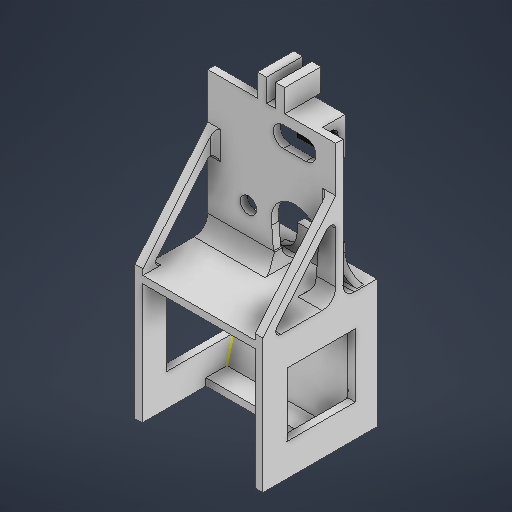
# Autodesk Inventor part: ведро
Saved by Autodesk Inventor 2025 (Build 290162000, 162)
## iProperties
Created: 2025-01-14
Part Number: ведро
Material: Типовые
Document SubType Name: Modeling
Designer: Phantom
Density: 1 g/cm^3
Appearance: По умолчанию
Author: Phantom
Autodesk Inventor part; units mm, degrees
ref_plane "YZ Plane" through (0, 0, 0) normal (1, 0, 0) x (0, 1, 0)
ref_plane "XZ Plane" through (0, 0, 0) normal (0, 1, 0) x (-1, 0, 0)
ref_plane "XY Plane" through (0, 0, 0) normal (0, 0, 1) x (1, 0, 0)
sketch "Эскиз9" plane through (0, 0, 0) normal (0, 0, 1) x (1, 0, 0)
  line L0 (-25, -25) -> (25, -25)
  line L1 (25, -25) -> (25, 25)
  line L2 (25, 25) -> (-25, 25)
  line L3 (-25, 25) -> (-25, -25)
  line L4 (-25, -25) -> (25, 25) construction
  line L5 (25, -25) -> (-25, 25) construction
  point P0 (0, 0)
  dimension "d29" = 50
  dimension "d30" = 50
  constraints: 12 end point, 2 midpoint, 2 parallel, 1 horizontal, 1 perpendicular
  measures "d29" distance of L2.end L1.end
  measures "d30" distance of L1.end L0.end
extrude "Выдавливание9" add sketch "Эскиз9" along normal blind 3.2
sketch "Эскиз10" plane through (0, 0, 0) normal (0, 0, -1) x (-1, 0, 0)
  line L0 (28.2, 28.2) -> (-28.2, 28.2)
  line L1 (-28.2, 28.2) -> (-28.2, -28.2)
  line L2 (-28.2, -28.2) -> (28.2, -28.2)
  line L3 (28.2, -28.2) -> (28.2, 28.2)
  line L4 (28.2, 28.2) -> (-28.2, -28.2) construction
  line L5 (-28.2, 28.2) -> (28.2, -28.2) construction
  line L6 (-25, -25) -> (-25, 25) projected
  line L7 (25, -25) -> (-25, -25) projected
  line L8 (25, 25) -> (25, -25) projected
  line L9 (-25, 25) -> (25, 25) projected
  point P0 (0, 0)
  dimension "d33" = 56.4
  dimension "d34" = 56.4
  constraints: 12 end point, 2 midpoint, 2 parallel, 1 horizontal, 1 perpendicular
  measures "d33" distance of L2.end L1.end
  measures "d34" distance of L1.end L0.end
extrude "Выдавливание10" add sketch "Эскиз10" against normal blind 47.2
sketch "Эскиз11" plane through (-28.2, -28.2, 0) normal (-1, 0, 0) x (0, 0, 1)
  line L0 (0, 56.4) -> (47.2, 56.4) projected
  line L1 (23.6, 56.4) -> (23.6, 0)
  line L2 (0, 0) -> (47.2, 0) projected
  line L3 (47.2, 53.2) -> (47.2, 3.2) projected
  line L4 (47.2, 28.2) -> (0, 28.2)
  line L5 (7.6, 42.2) -> (39.6, 42.2)
  line L6 (39.6, 42.2) -> (39.6, 14.2)
  line L7 (39.6, 14.2) -> (7.6, 14.2)
  line L8 (7.6, 14.2) -> (7.6, 42.2)
  line L9 (7.6, 42.2) -> (39.6, 14.2) construction
  line L10 (39.6, 42.2) -> (7.6, 14.2) construction
  line L11 (7.6, 42.2) -> (9.6, 42.2)
  line L12 (9.6, 42.2) -> (9.6, 0)
  point P0 (23.6, 28.2)
  point P1 (9.6, 14.2)
  dimension "d37" = 32
  dimension "d38" = 28
  dimension "d51" = 2
  constraints: 20 end point, 6 midpoint, 2 horizontal, 2 parallel, 2 perpendicular, 2 point on line
  measures "d37" distance of L6.end L7.end
  measures "d38" distance of L5.end L6.end
  measures "d51" distance of L5.start L11.end
extrude "Выдавливание11" cut sketch "Эскиз11" against normal through all contours L5 L6 L4 L1 | L1 L4 L12 L5 | L4 L6 L7 L1 | L1 L7 L12 L4
sketch "Эскиз12" plane through (0, 0, 47.2) normal (0, 0, 1) x (1, 0, 0)
  line L0 (28.2, -28.2) -> (28.2, 28.2) projected
  line L1 (28.2, 28.2) -> (-28.2, 28.2) projected
  line L2 (-28.2, 28.2) -> (-28.2, -28.2) projected
  line L3 (-28.2, -28.2) -> (28.2, -28.2) projected
  line L4 (25, 25) -> (25, -25) projected
  line L5 (25, -25) -> (-25, -25) projected
  line L6 (-25, -25) -> (-25, 25) projected
  line L7 (-25, 25) -> (25, 25) projected
  line L8 (25, -25) -> (25, -28.2)
  line L9 (-25, -25) -> (-25, -28.2)
  point P0 (0, 0)
  constraints: 4 end point, 2 perpendicular, 2 point on line
extrude "Выдавливание12" cut sketch "Эскиз12" against normal blind 25 contours L3 L9 L5 L8
sketch "Эскиз13" plane through (-25, -28.2, 47.2) normal (1, 0, 0) x (0, 0, -1)
  line L0 (37.6, 14.2) -> (7.6, 14.2) projected
  line L1 (7.6, 14.2) -> (7.6, 42.2) projected
  line L2 (7.6, 42.2) -> (37.6, 42.2) projected
  line L3 (44, 53.2) -> (44, 3.2) projected
  line L4 (44, 53.2) -> (0, 53.2) projected
  line L5 (0, 0) -> (0, 53.2) projected
  line L6 (25, 0) -> (0, 0) projected
  line L7 (25, 0) -> (25, 3.2) projected
  line L8 (44, 3.2) -> (25, 3.2) projected
  line L9 (0, 53.2) -> (44, 42.2)
  line L10 (44, 53.2) -> (44, 3.2) projected
  line L11 (37.6, 42.2) -> (37.6, 14.2) projected
  point P0 (47.2, 28.2)
  constraints: 2 end point, 1 point on line
extrude "Выдавливание13" add sketch "Эскиз13" along normal up to surface (50 mm away) contours L3 L9 L4
sketch "Эскиз14" plane through (-25, -28.2, 22.2) normal (1, 0, 0) x (0, 0, -1)
  line L0 (19, 42.2) -> (9, 2)
  line L1 (19, 42.2) -> (-25, 53.2) projected
  line L2 (-25, 0) -> (-25, 53.2) projected
  line L3 (0, 0) -> (-25, 0) projected
  line L4 (0, 0) -> (0, 3.2) projected
  line L5 (19, 3.2) -> (0, 3.2) projected
  line L6 (19, 42.2) -> (19, 3.2) projected
  line L7 (12.6, 14.2) -> (-17.4, 14.2) projected
  line L8 (-17.4, 14.2) -> (-17.4, 42.2) projected
  line L9 (-17.4, 42.2) -> (12.6, 42.2) projected
  line L10 (12.6, 42.2) -> (12.6, 14.2) projected
  point P0 (22.2, 28.2)
  point P1 (9.2985, 3.2)
  constraints: 2 end point
extrude "Выдавливание14" add sketch "Эскиз14" along normal up to surface (50 mm away) contours L6 L5 L0 L7 L10 | L10 L7 L0
sketch "Эскиз15" plane through (-25, -14, 39.6) normal (1, 0, 0) x (0, 0, -1)
  line L0 (30, 2.272) -> (36.4, 28) projected
  line L1 (-7.6, 39) -> (36.4, 28)
  line L2 (26.6985, -11) -> (29.4348, 0) projected
  line L3 (36.4, 28) -> (26.6985, -11)
  point P0 (39.6, 14)
  point P1 (32, 10.312)
  constraints: 4 end point
sketch "Эскиз16" plane through (-28.2, 28.2, 0) normal (0, 1, 0) x (1, 0, 0)
  line L0 (76, -15) -> (-29, -15)
  line L1 (0, 0) -> (56.4, 0) projected
  line L2 (3.2, -22.2) -> (53.2, -22.2) projected
  line L3 (0, 0) -> (56.4, 0) projected
  line L4 (0, 0) -> (0, -47.2) projected
  line L5 (56.4, -47.2) -> (0, -47.2) projected
  line L6 (56.4, 0) -> (56.4, -47.2) projected
  line L7 (77.0235, -18.2) -> (-32.0235, -18.2)
  point P0 (28.2, 0)
  point P1 (0, -18.2)
  point P2 (56.4, -18.2)
  point P3 (56.4, -15)
  point P4 (0, -15)
  dimension "d47" = 15
  dimension "d48" = 3.2
  constraints: 4 end point, 1 horizontal, 1 parallel
  measures "d47" distance between parallel lines of L1 L0
  measures "d48" distance between parallel lines of L0 L7
extrude "Выдавливание15" add sketch "Эскиз16" along normal blind 40 contours L6 L7 L4 L0
sketch "Эскиз17" plane through (28.2, 28.2, 15) normal (0, 0, -1) x (-1, 0, 0)
  line L0 (0, 40) -> (56.4, 40) projected
  line L1 (28.2, 40) -> (28.2, 0)
  line L2 (0, 0) -> (56.4, 0) projected
  line L3 (0, 0) -> (0, 40) projected
  line L4 (0, 18) -> (56.4, 18)
  circle A0 centre (17.95, 18) radius 3.6056
  circle A1 centre (38.45, 18) radius 3.6056
  point P0 (28.2, -28.2)
  point P1 (28.2, 18)
  dimension "d55" = 20.5
  dimension "d57" = 18
  constraints: 4 end point, 3 midpoint, 2 centre point, 2 point on line, 1 horizontal, 1 symmetric about line, 1 other
  measures "d55" distance of A1.centre A0.centre
  measures "d57" distance between parallel lines of L2 L4
extrude "Выдавливание16" cut sketch "Эскиз17" against normal blind 10 contours A0 L4 | L4 A0 | A1 L4 | L4 A1
sketch "Эскиз18" plane through (-28.2, 28.2, 18.2) normal (0, 0, 1) x (1, 0, 0)
  point P0 (28.2, -28.2)
sketch "Эскиз20" plane through (-28.2, 28.2, 18.2) normal (0, 0, 1) x (1, 0, 0)
  point P0 (28.2, -28.2)
sketch "Эскиз23" plane through (28.2, -28.2, 0) normal (1, 0, 0) x (0, 0, -1)
  line L0 (-18.2, 56.4) -> (-47.2, 56.4) projected
  line L1 (-47.2, 56.4) -> (-18.2, 91)
  line L2 (-18.2, 56.4) -> (-18.2, 96.4) projected
  line L3 (-47.2, 56.4) -> (-50.2656, 58.9694)
  line L4 (-50.2656, 58.9694) -> (-18.2, 97.227)
  line L5 (-50.2656, 58.9694) -> (-50.2656, 56.4)
  line L6 (-47.2, 56.4) -> (-50.2656, 56.4)
  line L7 (-18.2, 96.4) -> (-18.2, 97.227)
  line L8 (-18.2, 97.227) -> (-15, 97.227)
  line L9 (-15, 97.227) -> (-15, 96.4)
  line L10 (-39.6, 14.2) -> (-39.6, 42.2) projected
  line L11 (-39.6, 42.2) -> (-9.6, 42.2) projected
  line L12 (-9.6, 42.2) -> (-9.6, 14.2) projected
  line L13 (-9.6, 14.2) -> (-39.6, 14.2) projected
  line L14 (0, 56.4) -> (0, 0) projected
  line L15 (0, 56.4) -> (-15, 56.4) projected
  line L16 (-15, 56.4) -> (-15, 96.4) projected
  line L17 (-18.2, 96.4) -> (-15, 96.4) projected
  line L18 (-18.2, 56.4) -> (-18.2, 96.4) projected
  line L19 (-18.2, 56.4) -> (-47.2, 56.4) projected
  line L20 (-47.2, 0) -> (-47.2, 56.4) projected
  line L21 (0, 0) -> (-47.2, 0) projected
  point P0 (0, 28.2)
  dimension "d60" = 4
  constraints: 16 end point, 2 perpendicular, 2 vertical, 1 horizontal, 1 point on line, 1 other
  measures "d60" distance of L0.end L3.end
extrude "Выдавливание17" add sketch "Эскиз23" against normal blind 3.5 contours L3 L4 L7 L2 L1 | L6 L5 L3 | L7 L8 L9 L17
sketch "Эскиз24" plane through (0, 0, 47.2) normal (0, 0, 1) x (1, 0, 0)
  line L0 (-25, -28.2) -> (-25, 25) projected
  line L1 (25, 25) -> (25, -28.2) projected
  line L2 (25, -28.2) -> (28.2, -28.2) projected
  line L3 (28.2, -28.2) -> (28.2, 28.2) projected
  line L4 (28.2, 28.2) -> (24.7, 28.2) projected
  line L5 (-28.2, 28.2) -> (-28.2, -28.2) projected
  line L6 (-28.2, -28.2) -> (-25, -28.2) projected
  line L7 (-25, -28.2) -> (-25, 25) projected
  line L8 (-25, 25) -> (25, 25) projected
  line L9 (24.7, 28.2) -> (-28.2, 28.2) projected
  point P0 (0, 0)
extrude "Выдавливание18" add sketch "Эскиз24" along normal up to surface (3.0656 mm away)
fillet "Сопряжение1" radius 2.25 1 edges at (26.45, 28.2, 47.2)
sketch "Эскиз25" plane through (-28.2, -28.2, 0) normal (-1, 0, 0) x (0, 0, 1)
  line L0 (18.2, 91) -> (44.1028, 60.0953) projected
  arc A0 (42.3784, 56.4) -> (44.1028, 60.0953) centre (42.3784, 58.65) ccw projected
  line L1 (42.3784, 56.4) -> (50.2656, 56.4) projected
  line L2 (50.2656, 56.4) -> (50.2656, 58.9694) projected
  line L3 (50.2656, 58.9694) -> (18.2, 97.227) projected
  line L4 (18.2, 97.227) -> (15, 97.227) projected
  line L5 (15, 97.227) -> (15, 96.4) projected
  line L6 (18.2, 96.4) -> (15, 96.4) projected
  line L7 (18.2, 91) -> (18.2, 96.4) projected
  point P0 (0, 28.2)
extrude "Выдавливание19" add sketch "Эскиз25" against normal blind 3.5
sketch "Эскиз26" plane through (-28.2, 68.2, 0) normal (0, 1, 0) x (1, 0, 0)
  line L0 (3.5, -15) -> (3.5, -18.2) projected
  line L1 (3.5, -18.2) -> (52.9, -18.2) projected
  line L2 (52.9, -18.2) -> (52.9, -15) projected
  line L3 (52.9, -15) -> (3.5, -15) projected
  point P0 (28.2, 0)
extrude "Выдавливание20" add sketch "Эскиз26" along normal up to surface (0.827 mm away)
fillet "Сопряжение2" radius 2.25 3 edges at (-26.45, 62.8, 18.2) (26.45, 62.8, 18.2) (24.7, 65.9135, 18.2)
fillet "Сопряжение3" radius 2.25 2 edges at (-24.7, 65.9135, 18.2) (-24.7, 59.7064, 18.2)
sketch "Эскиз27" plane through (28.2, 69.027, 18.2) normal (0, 1, 0) x (1, 0, 0)
  line L0 (0, 3.2) -> (0, 0) projected
  line L1 (0, 3.2) -> (-56.4, 3.2) projected
  line L2 (-56.4, 0) -> (-56.4, 3.2) projected
  line L3 (-56.4, 0) -> (-50.65, 0) projected
  line L4 (-5.75, 0) -> (-50.65, 0) projected
  line L5 (0, 0) -> (-5.75, 0) projected
  point P0 (-28.2, 18.2)
extrude "Выдавливание21" add sketch "Эскиз27" along normal blind 20
sketch "Эскиз29" plane through (-28.2, 28.2, 18.2) normal (0, 0, 1) x (1, 0, 0)
  arc A0 (41.2392, 52.894) -> (45.2392, 52.9124) centre (43.2439, 51.8725) ccw projected
  arc A1 (31.3393, 52.8484) -> (35.3393, 52.8668) centre (33.3441, 51.8268) ccw projected
  arc A2 (45.4699, 2.8514) -> (41.4699, 2.833) centre (43.4652, 3.873) ccw projected
  arc A3 (35.57, 2.8058) -> (31.57, 2.7874) centre (33.5653, 3.8273) ccw projected
  circle A4 centre (33.5653, 3.8273) radius 2.25
  circle A5 centre (43.4652, 3.873) radius 2.25
  circle A6 centre (43.2439, 51.8725) radius 2.25
  circle A7 centre (33.3441, 51.8268) radius 2.25
  circle A8 centre (33.3441, 51.8268) radius 4.5
  circle A9 centre (43.2439, 51.8725) radius 4.5
  circle A10 centre (33.5653, 3.8273) radius 4.5
  circle A11 centre (43.4652, 3.873) radius 4.5
  line L0 (43.2439, 56.3725) -> (33.3233, 56.3268)
  line L1 (43.2439, 47.3725) -> (33.3648, 47.3269)
  line L2 (43.4239, 8.3728) -> (33.5445, 8.3273)
  line L3 (56.4, 0) -> (0, 0) projected
  point P0 (28.2, -28.2)
  point P1 (31.57, 2.7874)
  point P2 (35.57, 2.8058)
  point P3 (41.4699, 2.833)
  point P4 (45.4699, 2.8514)
  point P5 (45.2392, 52.9124)
  point P6 (41.2392, 52.894)
  point P7 (35.3393, 52.8668)
  point P8 (31.3393, 52.8484)
  point P9 (41.1738, 0)
  point P10 (31.1985, 0)
  point P11 (45.7565, 0)
  point P12 (43.2025, 56.3723)
  dimension "d93" = 9
  dimension "d94" = 9
  dimension "d91" = 9
  dimension "d92" = 9
  constraints: 8 coincident, 6 centre point, 6 end point, 4 point on circle, 3 concentric, 2 tangent, 7 other
  measures "d91" diameter of A8
  measures "d92" diameter of A9
extrude "Выдавливание22" cut sketch "Эскиз29" against normal blind 20 contours A6 A0 | A7 A1 | A5 A2 | A4 A3 | A8 | A8 L0 A9 L1 | A10 L3 | A10 L2 A11 L3 | A11 L3 picked at (33.4777, 0.5309) picked at (43.3776, 0.5461)
sketch "Эскиз30" plane through (28.2, 28.2, 15) normal (0, 0, -1) x (-1, 0, 0)
  line L0 (0, 60.827) -> (56.4, 60.827) projected
  line L1 (27, 60.827) -> (9, 60.827)
  line L2 (9, 60.827) -> (9, 57.627)
  line L3 (9, 57.627) -> (27, 57.627)
  line L4 (27, 57.627) -> (27, 60.827)
  point P0 (28.2, -28.2)
  point P1 (9, 60.827)
  dimension "d79" = 18
  dimension "d80" = 3.2
  constraints: 8 end point, 2 parallel, 1 horizontal, 1 perpendicular, 1 point on line
  measures "d79" distance of L3.end L2.end
  measures "d80" distance of L2.end L1.end
extrude "Выдавливание23" add sketch "Эскиз30" along normal blind 10
sketch "Эскиз31" plane through (1.2, 85.827, 15) normal (0, -1, 0) x (1, 0, 0)
  line L0 (0, 0) -> (0, -10) projected
  line L1 (0, -10) -> (18, -10)
  line L2 (18, -10) -> (18, -6.8)
  line L3 (18, -6.8) -> (0, -6.8)
  line L4 (0, -6.8) -> (0, -10)
  point P0 (-1.2, -15)
  point P1 (0, -6.8)
  dimension "d83" = 18
  dimension "d84" = 3.2
  constraints: 8 end point, 2 parallel, 1 horizontal, 1 perpendicular
  measures "d83" distance of L3.end L2.end
  measures "d84" distance of L2.end L1.end
extrude "Выдавливание24" add sketch "Эскиз31" along normal blind 13
sketch "Эскиз32" plane through (28.2, 28.2, 5) normal (0, 0, -1) x (-1, 0, 0)
  circle A0 centre (13.1561, 51.8725) radius 2.25 projected
  circle A1 centre (23.0559, 51.8268) radius 2.25 projected
  point P0 (28.2, -28.2)
extrude "Выдавливание25" cut sketch "Эскиз32" against normal blind 13
fillet "Сопряжение5" radius 3 1 edges at (10.2, 85.827, 8.2)
fillet "Сопряжение6" radius 6 2 edges at (22.8782, 28.2, 18.2) (-12.6007, 28.2, 18.2)
sketch "Эскиз33" plane through (28.2, 28.2, 5) normal (0, 0, -1) x (-1, 0, 0)
  arc A0 (12.9761, 8.3728) -> (10.6435, 0) centre (12.9348, 3.873) ccw projected
  circle A1 centre (12.9348, 3.873) radius 2.25
  arc A2 (25.2015, 0) -> (22.8555, 8.3273) centre (22.8347, 3.8273) ccw projected
  circle A3 centre (22.8347, 3.8273) radius 2.25
  circle A4 centre (13.1561, 51.8725) radius 2.25 projected
  circle A5 centre (23.0559, 51.8268) radius 2.25 projected
  line L0 (27, 60.827) -> (27, 44.627) projected
  line L1 (27, 60.827) -> (9, 60.827) projected
  line L2 (9, 60.827) -> (9, 44.627) projected
  line L3 (27, 44.627) -> (9, 44.627) projected
  line L4 (0, 6) -> (0, 28.4128) projected
  line L5 (56.4, 28.4128) -> (56.4, 30.6628) projected
  line L6 (0, 28.4128) -> (56.4, 28.4128)
  line L7 (27, -4.0014) -> (27, 12.1986)
  line L8 (27, -4.0014) -> (9, -4.0014)
  line L9 (9, -4.0014) -> (9, 12.1986)
  line L10 (27, 12.1986) -> (9, 12.1986)
  point P0 (28.2, -28.2)
  point P1 (56.4, 29.8581)
  dimension "d96" = 4.5
  dimension "d97" = 4.5
  constraints: 10 end point, 4 symmetric about line, 2 centre point, 2 coincident, 1 horizontal
  measures "d96" diameter of A1
  measures "d97" diameter of A3
extrude "Выдавливание26" add sketch "Эскиз33" against normal up to surface (3.2 mm away) contours L9 L10 L7 L8
fillet "Сопряжение7" radius 8.25 2 edges at (1.2, 28.2, 6.6) (19.2, 28.2, 6.6)
sketch "Эскиз34" plane through (28.2, 28.2, 15) normal (0, 0, -1) x (-1, 0, 0)
  circle A0 centre (18, 18) radius 10.5
  line L0 (26.7755, 6) -> (56.4, 6) projected
  circle A1 centre (38.45, 18) radius 3.6056 projected
  circle A2 centre (17.95, 18) radius 3.6056 projected
  line L1 (13.1975, 56.3723) -> (23.0767, 56.3268) projected
  arc A3 (23.0352, 47.3269) -> (23.0767, 56.3268) centre (23.0559, 51.8268) ccw projected
  line L2 (23.0352, 47.3269) -> (13.1561, 47.3725) projected
  arc A4 (13.1975, 56.3723) -> (13.1561, 47.3725) centre (13.1561, 51.8725) ccw projected
  line L3 (27, 57.627) -> (9, 57.627) projected
  line L4 (0, 60.827) -> (9, 60.827) projected
  line L5 (0, 0) -> (0, 60.827) projected
  line L6 (10.6435, 0) -> (0, 0) projected
  arc A5 (12.9761, 8.3728) -> (10.6435, 0) centre (12.9348, 3.873) ccw projected
  line L7 (12.9761, 8.3728) -> (22.8555, 8.3273) projected
  arc A6 (25.2015, 0) -> (22.8555, 8.3273) centre (22.8347, 3.8273) ccw projected
  line L8 (56.4, 0) -> (25.2015, 0) projected
  line L9 (56.4, 0) -> (56.4, 60.827) projected
  line L10 (27, 60.827) -> (56.4, 60.827) projected
  line L11 (28.2, 15.508) -> (27.3313, 4.0037)
  arc A7 (25.2015, 0) -> (22.8555, 8.3273) centre (22.8347, 3.8273) ccw projected
  line L12 (7.8, 15.508) -> (8.5999, 5.0806)
  line L13 (9, 57.627) -> (9, 60.827) projected
  line L14 (27, 60.827) -> (27, 57.627) projected
  point P0 (28.2, -28.2)
  point P1 (27.482, 6)
  dimension "d101" = 21
  constraints: 4 end point, 4 point on circle, 1 centre point
  measures "d101" diameter of A0
extrude "Выдавливание27" cut sketch "Эскиз34" against normal blind 10 contours A0 L7 | A0 L7 A5 L12 | L11 L0 A6 L7 A0 picked at (18.0986, 10.3735)
fillet "Сопряжение8" radius 7 1 edges at (-12.6007, 28.2, 15)
fillet "Сопряжение9" radius 5 1 edges at (22.8782, 28.2, 15)
sketch "Эскиз36" plane through (28.2, 89.027, 18.2) normal (0, 1, 0) x (1, 0, 0)
  line L0 (-7.5, 0) -> (-28.5, 0) projected
  line L1 (-28.5, 0) -> (-26.5, 0)
  line L2 (-26.5, 0) -> (-26.5, 16)
  line L3 (-26.5, 16) -> (-28.5, 16)
  line L4 (-28.5, 16) -> (-28.5, 0)
  line L5 (-26.5, 0) -> (-22.5, 0)
  line L6 (-22.5, 0) -> (-22.5, 16)
  line L7 (-22.5, 16) -> (-26.5, 16)
  line L8 (-26.5, 16) -> (-26.5, 0)
  line L9 (-28.5, 0) -> (-30.5, 0)
  line L10 (-30.5, 0) -> (-30.5, 16)
  line L11 (-30.5, 16) -> (-28.5, 16)
  line L12 (-28.5, 16) -> (-28.5, 0)
  line L13 (-30.5, 0) -> (-34.5, 0)
  line L14 (-34.5, 0) -> (-34.5, 16)
  line L15 (-34.5, 16) -> (-30.5, 16)
  line L16 (-30.5, 16) -> (-30.5, 0)
  point P0 (-28.2, 18.2)
  point P1 (-28.2, 0)
  point P2 (-7.8, 0)
  dimension "d113" = 2
  dimension "d114" = 4
  dimension "d115" = 2
  dimension "d116" = 4
  constraints: 32 end point, 8 parallel, 4 horizontal, 4 perpendicular, 3 point on line
  measures "d113" distance of L3.end L2.end
  measures "d114" distance of L7.end L6.end
  measures "d115" distance of L10.end L11.end
  measures "d116" distance of L14.end L15.end
extrude "Выдавливание29" add sketch "Эскиз36" along normal blind 10 contours L0 L2 L7 L6 | L13 L14 L15 L10
